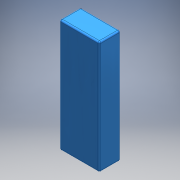
# Autodesk Inventor part: battery_model
Saved by Autodesk Inventor 2016 (Build 200138000, 138)
## iProperties
Created: 2016-03-07
Part Number: battery_model
Material: Generic
Document SubType Name: Modeling
Designer: dimas
Density: 1 g/cm^3
Appearance: Cyan
Author: dimas
Autodesk Inventor part; units mm, degrees
ref_plane "YZ Plane" through (0, 0, 0) normal (1, 0, 0) x (0, 1, 0)
ref_plane "XZ Plane" through (0, 0, 0) normal (0, 1, 0) x (-1, 0, 0)
ref_plane "XY Plane" through (0, 0, 0) normal (0, 0, 1) x (1, 0, 0)
sketch "Sketch1" plane through (0, 0, 0) normal (0, 1, 0) x (-1, 0, 0)
  line L0 (0, 0) -> (51, 0)
  line L1 (51, 0) -> (51, 144)
  line L2 (51, 144) -> (0, 144)
  line L3 (0, 144) -> (0, 0)
  dimension "d0" = 51
  dimension "d1" = 144
  constraints: 8 end point, 2 parallel, 1 horizontal, 1 perpendicular
  measures "d0" distance of L2.end L1.end
  measures "d1" distance of L1.end L0.end
extrude "Extrusion1" add sketch "Sketch1" along normal blind 27
fillet "Fillet1" radius 2 12 edges at (-25.5, 27, 144) (0, 27, 72) (-51, 27, 72) (-25.5, 27, 0) (-25.5, 0, 144) (0, 0, 72) (-25.5, 0, 0) (-51, 0, 72) (0, 13.5, 0) (0, 13.5, 144) (-51, 13.5, 144) (-51, 13.5, 0)
body "Solid1"
